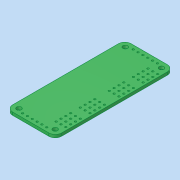
# Autodesk Inventor part: MainPCB
Saved by Autodesk Inventor 2017 (Build 210142000, 142)
## iProperties
Created: 2017-01-25
Part Number: MainPCB
Material: Silicon Nitride
Document SubType Name: Modeling
Designer: techn
Density: 3.18 g/cm^3
Appearance: Flaked Satin - Sea Green
Mass: 7.35571 g
Surface Area: 36.3647 cm^2
Volume: 2.31312 cm^3
Author: techn
Autodesk Inventor part; units mm, degrees
ref_plane "YZ Plane" through (0, 0, 0) normal (1, 0, 0) x (0, 1, 0)
ref_plane "XZ Plane" through (0, 0, 0) normal (0, 1, 0) x (-1, 0, 0)
ref_plane "XY Plane" through (0, 0, 0) normal (0, 0, 1) x (1, 0, 0)
sketch "Sketch1" plane through (0, 0, 0) normal (0, 1, 0) x (-1, 0, 0)
  line L0 (0, 0) -> (25.654, 0)
  line L1 (25.654, 0) -> (25.654, -62.23)
  line L2 (25.654, -62.23) -> (0, -62.23)
  line L3 (0, -62.23) -> (0, 0)
  circle A0 centre (3.302, -3.302) radius 1.27
  circle A1 centre (3.302, -59.182) radius 1.27
  circle A2 centre (22.352, -3.302) radius 1.27
  circle A3 centre (22.352, -59.182) radius 1.27
  dimension "d0" = 25.654
  dimension "d1" = 2.54
  dimension "d2" = 3.302
  dimension "d3" = 3.302
  dimension "d4" = 62.23
  dimension "d7" = 55.88
  dimension "d10" = 19.05
  constraints: 8 end point, 4 centre point, 2 horizontal, 2 parallel, 1 perpendicular, 1 vertical, 6 other
  measures "d0" distance of L1.end L2.end
  measures "d1" diameter of A0
  measures "d2" distance from line of A0.centre L3
  measures "d3" distance from line of A0.centre L0
  measures "d4" distance of L0.end L1.end
  measures "d7" distance of A0.centre A1.centre
  measures "d10" distance of A0.centre A2.centre
extrude "Extrusion1" add sketch "Sketch1" along normal blind 1.524
sketch "Sketch2" plane through (0, 1.524, 0) normal (0, 1, 0) x (1, 0, 0)
  circle A0 centre (-19.177, 2.032) radius 0.51
  line L0 (-25.654, 0) -> (0, 0) projected
  circle A1 centre (-16.637, 2.032) radius 0.51
  circle A2 centre (-14.097, 2.032) radius 0.51
  circle A3 centre (-11.557, 2.032) radius 0.51
  circle A4 centre (-9.017, 2.032) radius 0.51
  circle A5 centre (-6.477, 2.032) radius 0.51
  circle A6 centre (-22.352, 3.302) radius 1.27 projected
  circle A7 centre (-6.604, 7.112) radius 0.51
  line L1 (-25.654, 62.23) -> (-25.654, 0) projected
  circle A8 centre (-6.604, 9.652) radius 0.51
  circle A9 centre (-6.604, 12.192) radius 0.51
  circle A10 centre (-6.604, 14.732) radius 0.51
  circle A11 centre (-4.064, 7.112) radius 0.51
  circle A12 centre (-4.064, 9.652) radius 0.51
  circle A13 centre (-4.064, 12.192) radius 0.51
  circle A14 centre (-4.064, 14.732) radius 0.51
  circle A15 centre (-1.524, 7.112) radius 0.51
  circle A16 centre (-1.524, 9.652) radius 0.51
  circle A17 centre (-1.524, 12.192) radius 0.51
  circle A18 centre (-1.524, 14.732) radius 0.51
  circle A19 centre (-3.302, 3.302) radius 1.27 projected
  line L2 (0, 0) -> (0, 62.23) projected
  circle A20 centre (-4.064, 19.812) radius 0.51
  circle A21 centre (-1.524, 19.812) radius 0.51
  circle A22 centre (-1.524, 22.352) radius 0.51
  circle A23 centre (-6.604, 24.892) radius 0.51
  circle A24 centre (-4.064, 24.892) radius 0.51
  circle A25 centre (-1.524, 24.892) radius 0.51
  circle A26 centre (-6.604, 27.432) radius 0.51
  circle A27 centre (-4.064, 27.432) radius 0.51
  circle A28 centre (-1.524, 27.432) radius 0.51
  circle A29 centre (-6.604, 22.352) radius 0.51
  circle A30 centre (-4.064, 22.352) radius 0.51
  circle A31 centre (-6.604, 19.812) radius 0.51
  circle A32 centre (-1.524, 37.592) radius 0.51
  circle A33 centre (-4.064, 37.592) radius 0.51
  circle A34 centre (-6.604, 37.592) radius 0.51
  circle A35 centre (-1.524, 40.132) radius 0.51
  circle A36 centre (-4.064, 40.132) radius 0.51
  circle A37 centre (-6.604, 40.132) radius 0.51
  circle A38 centre (-1.524, 42.672) radius 0.51
  circle A39 centre (-4.064, 42.672) radius 0.51
  circle A40 centre (-6.604, 42.672) radius 0.51
  circle A41 centre (-4.064, 35.052) radius 0.51
  circle A42 centre (-1.524, 35.052) radius 0.51
  circle A43 centre (-6.604, 35.052) radius 0.51
  circle A44 centre (-4.064, 47.752) radius 0.51
  circle A45 centre (-1.524, 47.752) radius 0.51
  circle A46 centre (-6.604, 47.752) radius 0.51
  circle A47 centre (-4.064, 50.292) radius 0.51
  circle A48 centre (-6.604, 50.292) radius 0.51
  circle A49 centre (-1.524, 50.292) radius 0.51
  circle A50 centre (-4.064, 52.832) radius 0.51
  circle A51 centre (-6.604, 52.832) radius 0.51
  circle A52 centre (-1.524, 52.832) radius 0.51
  circle A53 centre (-6.604, 55.372) radius 0.51
  circle A54 centre (-4.064, 55.372) radius 0.51
  circle A55 centre (-1.524, 55.372) radius 0.51
  circle A56 centre (-6.477, 60.198) radius 0.51
  circle A57 centre (-9.017, 60.198) radius 0.51
  circle A58 centre (-11.557, 60.198) radius 0.51
  circle A59 centre (-19.177, 60.198) radius 0.51
  circle A60 centre (-16.637, 60.198) radius 0.51
  circle A61 centre (-14.097, 60.198) radius 0.51
  dimension "d15" = 1.02
  dimension "d16" = 2.032
  dimension "d19" = 2.54
  dimension "d24" = 3.175
  dimension "d25" = 1.02
  dimension "d28" = 2.54
  dimension "d31" = 2.54
  dimension "d34" = 4.064
  dimension "d35" = 9.652
  dimension "d38" = 12.7
  dimension "d45" = 15.24
  dimension "d52" = 12.7
  dimension "d63" = 58.166
  constraints: 60 centre point, 5 vertical, 2 horizontal, 116 other
  measures "d15" diameter of A0
  measures "d16" distance from line of A0.centre L0
  measures "d19" distance of A0.centre A1.centre
  measures "d24" horizontal distance of A0.centre A6.centre
  measures "d25" diameter of A7
  measures "d28" distance of A7.centre A8.centre
  measures "d31" distance of A7.centre A11.centre
  measures "d34" distance from line of L2 A11.centre
  measures "d35" distance from line of A12.centre L0
  measures "d38" distance of A15.centre A21.centre
  measures "d45" distance of A22.centre A32.centre
  measures "d52" distance of A42.centre A45.centre
  measures "d63" distance of A0.centre A59.centre
extrude "Extrusion4" cut sketch "Sketch2" against normal through all contours A0 | A1 | A2 | A3 | A4 | A5 | A7 | A8 | A9 | A10 | A11 | A12 | A13 | A14 | A15 | A16 | A17 | A18 | A20 | A21 | A22 | A23 | A24 | A25 | A26 | A27 | A28 | A29 | A30 | A31 | A32 | A33 | A34 | A35 | A36 | A37 | A38 | A39 | A40 | A41 | A42 | A43 | A44 | A45 | A46 | A47 | A48 | A49 | A50 | A51 | A52 | A53 | A54 | A55 | A56 | A57 | A58 | A59 | A60 | A61
fillet "Fillet1" radius 3.302 4 edges at (-25.654, 0.762, 0) (0, 0.762, 0) (0, 0.762, -62.23) (-25.654, 0.762, -62.23)
body "Solid1"
